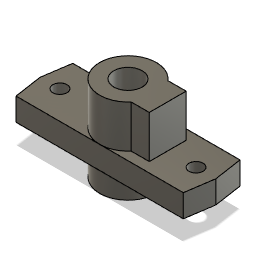
6432106821_NCV_11 (Autodesk Fusion 360 design; units mm, degrees)
Autodesk Fusion 360 part; units mm, degrees
note: some values were not read from the file. Set by a fixed rule: which sketch regions a step uses.
sketch "Sketch1" plane through (0, 0, 0) normal (0, 1, 0) x (1, 0, 0)
  line L0 (0, 0) -> (124, 0)
  line L1 (124, 0) -> (124, 40)
  line L2 (124, 40) -> (0, 40)
  line L3 (0, 40) -> (0, 0)
  circle A0 centre (14, 20) radius 5
  circle A1 centre (110, 20) radius 5
  line L4 (0, 20) -> (3, 0)
  line L5 (0, 20) -> (3, 40)
  line L6 (124, 20) -> (121, 0)
  line L7 (124, 20) -> (121, 40)
  circle A2 centre (62, 20) radius 20
  circle A3 centre (62, 20) radius 10
  line L8 (62, 33) -> (90, 33)
  line L9 (90, 33) -> (90, 7)
  line L10 (90, 7) -> (62, 7)
  line L11 (62, 7) -> (62, 33)
  dimension "d1" = 124
  dimension "d2" = 40
  dimension "d3" = 14
  dimension "d4" = 14
  dimension "d5" = 3
  dimension "d6" = 3
  dimension "d7" = 3
  dimension "d8" = 3
  dimension "d9" = 40
  dimension "d10" = 62
  dimension "d11" = 20
  dimension "d12" = 28
  dimension "d13" = 26
  dimension "d14" = 13
  dimension "d15" = 28
  constraint horizontal L0
  constraint vertical L1
  constraint horizontal L2
  constraint vertical L3
  constraint coincident L0.start L3.end
  constraint midpoint L3 L4.start
  constraint coincident L0 L4.end
  constraint coincident L2 L5.end
  constraint midpoint L1 L6.start
  constraint coincident L0 L6.end
  constraint coincident L2 L7.end
  constraint concentric A2 A3
  constraint horizontal L8
  constraint vertical L9
  constraint horizontal L10
  constraint vertical L11
  measures "d1" distance of L0.start L0.end
  measures "d2" distance of L0.start L2.end
  measures "d3" distance of L3 A0.centre
  measures "d4" distance of L1 A1.centre
  measures "d5" distance of L0.start L4.end
  measures "d6" distance of L2.end L5.end
  measures "d7" distance of L0.end L6.end
  measures "d8" distance of L1.end L7.end
  measures "d9" diameter of A2
  measures "d10" distance of L6.start A2.centre
  measures "d11" diameter of A3
  measures "d12" distance of L8.start L8.end
  measures "d13" distance of L8.start L10.end
  measures "d14" distance of A2.centre L8.start
  measures "d15" distance of A2.centre L9
extrude "Extrude1" add sketch "Sketch1" along normal blind 16 contours L0 L2 L4 L5 A2 | L0 L2 L6 L7 A2 L8 L9 L10
extrude "Extrude2" add sketch "Sketch1" along normal blind 46 contours A2 A3 L8 L10 L11 | A2 A3 L8 L10 L11 | A2 L8 L9 L10
extrude "Extrude3" add sketch "Sketch1" against normal blind 14 contours A2 A3 L8 L10 L11 | A2 A3 L8 L10 L11
equation "d10 = ( 124 / 2 ) * 1 mm"
